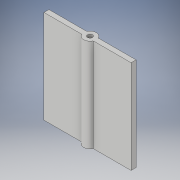
# Autodesk Inventor part: doughvpush
Saved by Autodesk Inventor 2019 (Build 230136000, 136)
## iProperties
Created: 2020-02-19
Part Number: doughvpush
Material: Generic
Document SubType Name: Modeling
Designer: ACHYUTH
Density: 1 g/cm^3
Appearance: Default
Author: ACHYUTH
Autodesk Inventor part; units mm, degrees
ref_plane "YZ Plane" through (0, 0, 0) normal (1, 0, 0) x (0, 1, 0)
ref_plane "XZ Plane" through (0, 0, 0) normal (0, 1, 0) x (-1, 0, 0)
ref_plane "XY Plane" through (0, 0, 0) normal (0, 0, 1) x (1, 0, 0)
sketch "Sketch1" plane through (0, 0, 0) normal (0, 1, 0) x (-1, 0, 0)
  circle A0 centre (0, 0) radius 5
  dimension "d0" = 10
  constraints: 1 centre point, 1 coincident
  measures "d0" diameter of A0
extrude "Extrusion1" add sketch "Sketch1" along normal mid plane 75
sketch "Sketch2" plane through (0, 0, 0) normal (1, 0, 0) x (0, 1, 0)
  line L0 (37.5, -5) -> (37.5, 5) projected
  line L1 (37.5, 0) -> (37.5, 2)
  line L2 (37.5, 2) -> (37.5, -2)
  line L3 (37.5, 2) -> (-37.5, 2)
  line L4 (-37.5, 2) -> (-37.5, -2)
  line L5 (-37.5, -2) -> (37.5, -2)
  line L6 (37.5, -2) -> (37.5, 2)
  point P0 (0, 0)
  dimension "d4" = 4
  dimension "d5" = 75
  constraints: 12 end point, 2 parallel, 2 point on line, 1 horizontal, 1 midpoint, 1 perpendicular
  measures "d4" distance of L1.end L2.end
  measures "d5" distance of L5.end L4.end
sketch "Sketch3" plane through (0, 0, 0) normal (1, 0, 0) x (0, 1, 0)
  point P0 (0, 0)
extrude "Extrusion2" add sketch "Sketch2" along normal mid plane 70
sketch "Sketch4" plane through (0, 37.5, 0) normal (0, 1, 0) x (1, 0, 0)
  point P0 (0, 0)
hole "Hole1" at (0, 37.5, 0) direction (0, -1, 0) diameter 4 depth 120
body "Solid1"
